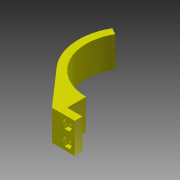
# Autodesk Inventor part: clip
Saved by Autodesk Inventor 2013 (Build 170138000, 138)
## iProperties
Created: 2013-12-08
Part Number: clip
Material: Generic
Document SubType Name: Modeling
Designer: employee
Density: 1 g/cm^3
Author: employee
Autodesk Inventor part; units mm, degrees
ref_plane "YZ Plane" through (0, 0, 0) normal (1, 0, 0) x (0, 1, 0)
ref_plane "XZ Plane" through (0, 0, 0) normal (0, 1, 0) x (-1, 0, 0)
ref_plane "XY Plane" through (0, 0, 0) normal (0, 0, 1) x (1, 0, 0)
sketch "Sketch1" plane through (0, 0, 0) normal (0, 0, 1) x (1, 0, 0)
  arc A0 (-30.4516, 17.5812) -> (0, -35.1625) centre (0, 0) ccw
  line L0 (0, 0) -> (30.1625, 0)
  line L1 (0, 0) -> (17.5813, 30.4516)
  line L2 (0, 0) -> (-30.4516, 17.5812)
  line L3 (0, -30.1625) -> (0, -35.1625)
  arc A1 (-26.1215, 15.0812) -> (0, -30.1625) centre (0, 0) ccw
  arc A2 (30.1625, 0) -> (15.0813, 26.1215) centre (0, 0) ccw
  line L4 (0, -30.1625) -> (30.1625, -30.1625)
  line L5 (30.1625, -30.1625) -> (30.1625, -42.6625)
  line L6 (30.1625, -42.6625) -> (0, -42.6625)
  line L7 (0, -42.6625) -> (0, -30.1625)
  line L8 (0, -42.6625) -> (10, -42.6625)
  line L9 (10, -42.6625) -> (10, -47.6625)
  line L10 (10, -47.6625) -> (0, -47.6625)
  line L11 (0, -47.6625) -> (0, -42.6625)
  line L12 (0, -47.6625) -> (0, -35.1625)
  line L13 (0, -47.6625) -> (-5, -47.6625)
  line L14 (-5, -47.6625) -> (-5, -42.6625)
  line L15 (-5, -42.6625) -> (0, -42.6625)
  line L16 (0, -42.6625) -> (0, -47.6625)
  line L17 (-5, -47.6625) -> (-26.4528, -23.1657)
  line L18 (0, -42.6625) -> (0, -35.1625)
  dimension "d3" = 60
  dimension "d4" = 30.1625
  dimension "d5" = 35.1625
  dimension "d6" = 12.5
  dimension "d7" = 10
  dimension "d8" = 5
  constraints: 38 end point, 7 point on circle, 6 parallel, 6 perpendicular, 4 horizontal, 3 centre point, 2 collinear, 2 point on line, 1 coincident, 1 concentric, 1 tangent, 1 vertical alignment
  measures "d3" angle of L0 L1
  measures "d4" radius of A1
  measures "d5" radius of A0
  measures "d6" distance between parallel lines of L4 L6
  measures "d7" distance of L9.end L10.end
  measures "d8" distance of L8.end L9.end
extrude "Extrusion1" add sketch "Sketch1" along normal blind 20 contours L2 A1 L3 A0 | A0 L7 L15 L14 L17 | L14 L15 L11 L13 | L6 L9 L10 L11
sketch "Sketch2" plane through (-5, -47.6625, 0) normal (0, -1, 0) x (1, 0, 0)
  line L0 (0, 0) -> (15, 0) projected
  line L1 (15, 0) -> (15, 20) projected
  line L2 (0, 20) -> (15, 20) projected
  line L3 (0, 0) -> (0, 20) projected
  line L4 (10, 20) -> (10, 0)
  circle A0 centre (10, 15) radius 1.6
  circle A1 centre (10, 5) radius 1.6
  point P0 (5, 0)
  dimension "d11" = 3.2
  dimension "d13" = 5
  dimension "d14" = 5
  dimension "d15" = 5
  constraints: 4 point on line, 2 centre point, 2 end point, 1 equal radius, 1 parallel
  measures "d11" diameter of A1
  measures "d13" distance from line of L2 A0.centre
  measures "d14" distance from line of L0 A1.centre
  measures "d15" distance between parallel lines of L1 L4
extrude "Extrusion2" cut sketch "Sketch2" against normal through all contours A1 L4 | L4 A1 | A0 L4 | L4 A0
sketch "Sketch3" plane through (-5, -47.6625, 0) normal (0, -1, 0) x (1, 0, 0)
  circle A0 centre (10, 5) radius 1.6 projected
  circle A1 centre (10, 15) radius 1.6 projected
  line L0 (6.738, 15) -> (8.369, 17.825)
  line L1 (8.369, 17.825) -> (11.631, 17.825)
  line L2 (11.631, 17.825) -> (13.262, 15)
  line L3 (13.262, 15) -> (11.631, 12.175)
  line L4 (11.631, 12.175) -> (8.369, 12.175)
  line L5 (8.369, 12.175) -> (6.738, 15)
  line L6 (6.738, 5) -> (8.369, 7.825)
  line L7 (8.369, 7.825) -> (11.631, 7.825)
  line L8 (11.631, 7.825) -> (13.262, 5)
  line L9 (13.262, 5) -> (11.631, 2.175)
  line L10 (11.631, 2.175) -> (8.369, 2.175)
  line L11 (8.369, 2.175) -> (6.738, 5)
  point P0 (5, 0)
  dimension "d18" = 5.65
  constraints: 24 end point, 2 coincident, 2 horizontal, 1 parallel, 26 other
  measures "d18" distance between parallel lines of L10 L7
extrude "Extrusion3" cut sketch "Sketch3" against normal blind 2.5
body "Solid1"
